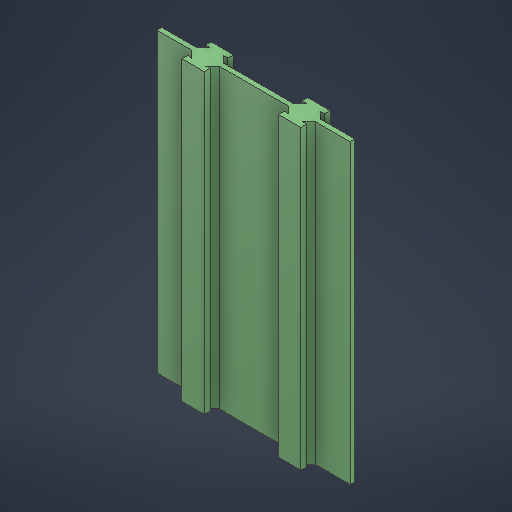
# Autodesk Inventor part: connector
Saved by Autodesk Inventor 2027 (Build 310192060, 192F)
## iProperties
Created: 2026-06-08
Part Number: connector
Material: Ogólny
Document SubType Name: Modeling
Designer: User
Density: 1 g/cm^3
Appearance: Domyślna
Author: User
Autodesk Inventor part; units mm, degrees
ref_plane "YZ Plane" through (0, 0, 0) normal (1, 0, 0) x (0, 1, 0)
ref_plane "XZ Plane" through (0, 0, 0) normal (0, 1, 0) x (-1, 0, 0)
ref_plane "XY Plane" through (0, 0, 0) normal (0, 0, 1) x (1, 0, 0)
sketch "Szkic1" plane through (0, 0, 0) normal (0, 1, 0) x (-1, 0, 0)
  line L0 (20.6403, -1) -> (18.625, -3.0153)
  line L1 (18.625, -3.0153) -> (20.05, -3.0153)
  line L2 (20.05, -3.0153) -> (20.05, -4.9153)
  line L3 (20.05, -4.9153) -> (16.25, -4.9153)
  line L4 (16.25, -4.9153) -> (16.25, -0.7939) construction
  line L5 (11.8597, -1) -> (13.875, -3.0153)
  line L6 (12.45, -4.9153) -> (16.25, -4.9153)
  line L7 (12.45, -3.0153) -> (12.45, -4.9153)
  line L8 (13.875, -3.0153) -> (12.45, -3.0153)
  line L9 (-32.5, 1) -> (32.5, 1)
  line L10 (32.5, 1) -> (32.5, -1)
  line L11 (32.5, -1) -> (-32.5, -1)
  line L12 (-32.5, -1) -> (-32.5, 1)
  line L13 (-32.5, 1) -> (32.5, -1) construction
  line L14 (32.5, 1) -> (-32.5, -1) construction
  line L15 (0, 0) -> (0, -5.7092) construction
  line L16 (0, 0) -> (5.7092, 0) construction
  line L17 (0, -2.8546) -> (16.25, -2.8546) construction
  line L18 (0, -2.8546) -> (16.25, -2.8546) construction
  line L19 (16.25, -0.7939) -> (16.25, -4.9153) construction
  line L20 (32.5, 0) -> (-32.5, 0) construction
  line L21 (-20.6403, -1) -> (-18.625, -3.0153)
  line L22 (-18.625, -3.0153) -> (-20.05, -3.0153)
  line L23 (-20.05, -3.0153) -> (-20.05, -4.9153)
  line L24 (-16.25, -4.9153) -> (-16.25, -0.7939) construction
  line L25 (-12.45, -3.0153) -> (-12.45, -4.9153)
  line L26 (-13.875, -3.0153) -> (-12.45, -3.0153)
  line L27 (-11.8597, -1) -> (-13.875, -3.0153)
  line L28 (-20.05, -4.9153) -> (-16.25, -4.9153)
  line L29 (-12.45, -4.9153) -> (-16.25, -4.9153)
  line L30 (0, -2.8546) -> (-16.25, -2.8546) construction
  line L31 (0, -2.8546) -> (-16.25, -2.8546) construction
  line L32 (-16.25, -0.7939) -> (-16.25, -4.9153) construction
  line L33 (20.6403, 1) -> (18.625, 3.0153)
  line L34 (18.625, 3.0153) -> (20.05, 3.0153)
  line L35 (20.05, 3.0153) -> (20.05, 4.9153)
  line L36 (16.25, 4.9153) -> (16.25, 0.7939) construction
  line L37 (12.45, 3.0153) -> (12.45, 4.9153)
  line L38 (13.875, 3.0153) -> (12.45, 3.0153)
  line L39 (11.8597, 1) -> (13.875, 3.0153)
  line L40 (20.05, 4.9153) -> (16.25, 4.9153)
  line L41 (12.45, 4.9153) -> (16.25, 4.9153)
  line L42 (0, 2.8546) -> (16.25, 2.8546) construction
  line L43 (0, 2.8546) -> (16.25, 2.8546) construction
  line L44 (16.25, 0.7939) -> (16.25, 4.9153) construction
  line L45 (-13.875, 3.0153) -> (-12.45, 3.0153)
  line L46 (-12.45, 3.0153) -> (-12.45, 4.9153)
  line L47 (-11.8597, 1) -> (-13.875, 3.0153)
  line L48 (0, 2.8546) -> (-16.25, 2.8546) construction
  line L49 (0, 2.8546) -> (-16.25, 2.8546) construction
  line L50 (-16.25, 4.9153) -> (-16.25, 0.7939) construction
  line L51 (-16.25, 0.7939) -> (-16.25, 4.9153) construction
  line L52 (-18.625, 3.0153) -> (-20.05, 3.0153)
  line L53 (-20.05, 3.0153) -> (-20.05, 4.9153)
  line L54 (-20.6403, 1) -> (-18.625, 3.0153)
  line L55 (-20.05, 4.9153) -> (-16.25, 4.9153)
  line L56 (-12.45, 4.9153) -> (-16.25, 4.9153)
  point P0 (0, -1)
  point P1 (-20.6403, 1)
  point P2 (-20.6403, -1)
  point P3 (-11.8597, -1)
  point P4 (13.4887, -1)
  point P5 (20.6403, -1)
  point P6 (20.6403, 1)
  point P7 (11.8597, 1)
  point P8 (-11.8597, 1)
  dimension "d20" = 2.85
  dimension "d21" = 1.425
  dimension "d22" = 1.9
  dimension "d23" = 3.8
  dimension "d24" = 45
  dimension "d25" = 65
  dimension "d26" = 2
  dimension "d32" = 90
  dimension "d33" = 16.25
  dimension "d34" = 0
  dimension "d35" = 1.8546
  constraints: 114 end point, 40 symmetric about line, 7 midpoint, 5 horizontal, 4 parallel, 3 vertical, 2 equal length, 2 perpendicular, 1 point on line
  measures "d20" distance of L0.start L0.end
  measures "d21" distance of L0.end L1.end
  measures "d22" distance of L1.end L2.end
  measures "d23" distance of L2.end L4.start
  measures "d24" angle of L8 L5
  measures "d25" distance of L10.end L11.end
  measures "d26" distance of L9.end L10.end
  measures "d32" angle of L15 L16
  measures "d33" distance of L17.end L17.start
  measures "d34" distance between parallel lines of L17 L18
  measures "d35" distance of point (0, -1) L17.start
extrude "Wyciągnięcie proste1" add sketch "Szkic1" along normal blind 100
offset faces "Rozmiar1" outward -0.2 faces at (-24.5935, 33.3333, -1) (3.9532, 33.3333, -1) (28.5468, 33.3333, -1) (24.5935, 33.3333, 1) (-3.9532, 33.3333, 1) (-28.5468, 66.6667, 1)
equation "\"d20\" = 3 * Scaller"
equation "\"d21\" = 1.5 * Scaller"
equation "\"d22\" = 2 * Scaller"
equation "\"d23\" = 4 * Scaller"
equation "\"Scaller\" = 0.95"
